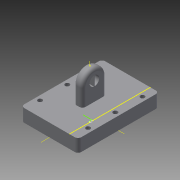
# Autodesk Inventor part: Camera holder with suppor final
Saved by Autodesk Inventor 2015 (Build 190159000, 159)
## iProperties
Created: 2016-05-06
Part Number: Camera holder with suppor final
Material: Generic
Document SubType Name: Modeling
Designer: Cristi
Density: 1 g/cm^3
Appearance: Default
Author: Cristi
Autodesk Inventor part; units mm, degrees
ref_plane "YZ Plane" through (0, 0, 0) normal (1, 0, 0) x (0, 1, 0)
ref_plane "XZ Plane" through (0, 0, 0) normal (0, 1, 0) x (-1, 0, 0)
ref_plane "XY Plane" through (0, 0, 0) normal (0, 0, 1) x (1, 0, 0)
sketch "Sketch1" plane through (0, 0, 0) normal (0, 0, 1) x (1, 0, 0)
  point P0 (0, 0)
sketch "Sketch2" plane through (0, 0, 0) normal (0, 1, 0) x (-1, 0, 0)
  line L0 (-17.8, 25.3) -> (-17.8, -25.3)
  line L1 (-17.8, -25.3) -> (-12.3, -25.3)
  line L2 (-12.3, -25.3) -> (-12.3, 25.3)
  line L3 (-12.3, 25.3) -> (-17.8, 25.3)
  circle A0 centre (-15, 16.2) radius 1.35
  circle A1 centre (-15, -0.8) radius 1.35
  circle A2 centre (-15, -17.8) radius 1.35
  point P0 (0, 0)
  point P1 (-17.8, 0)
  dimension "d0" = 50.6
  dimension "d1" = 5.5
  dimension "d2" = 2.8
  dimension "d3" = 2.7
  dimension "d4" = 9.1
  dimension "d5" = 2.7
  dimension "d6" = 2.7
  dimension "d7" = 17
  dimension "d8" = 17
  constraints: 8 end point, 3 centre point, 3 perpendicular, 2 vertical alignment, 1 midpoint, 1 vertical
  measures "d0" distance of L0.start L0.end
  measures "d1" distance of L0.end L1.end
  measures "d2" distance from line of L0 A0.centre
  measures "d3" diameter of A0
  measures "d4" distance from line of L3 A0.centre
  measures "d5" diameter of A1
  measures "d6" diameter of A2
  measures "d7" distance of A1.centre A2.centre
  measures "d8" distance of A0.centre A1.centre
extrude "Extrusion1" add sketch "Sketch2" along normal blind 8
sketch "Sketch3" plane through (12.3, 0, -25.3) normal (-1, 0, 0) x (0, 0, 1)
  line L0 (0, 8) -> (50.6, 8)
  line L1 (50.6, 8) -> (0, 8) projected
  line L2 (50.6, 8) -> (50.6, 5)
  line L3 (50.6, 0) -> (50.6, 8) projected
  line L4 (50.6, 5) -> (0, 5)
  line L5 (0, 0) -> (0, 8) projected
  point P0 (25.3, 0)
  dimension "d11" = 3
  constraints: 6 end point, 2 point on line, 1 collinear, 1 perpendicular
  measures "d11" distance of L0.end L2.end
extrude "Extrusion2" add sketch "Sketch3" along normal blind 12.3
mirror "Mirror1" about plane through (0, 0, 0) normal (1, 0, 0) of "Extrusion1", "Extrusion2"
sketch "Sketch4" plane through (0, 8, 0) normal (0, 1, 0) x (1, 0, 0)
  point P0 (0, 0)
sketch "Sketch5" plane through (0, 8, 0) normal (0, 1, 0) x (1, 0, 0)
  line L0 (-2.75, -7.5) -> (-2.75, 7.5)
  line L1 (-2.75, 7.5) -> (2.75, 7.5)
  line L2 (2.75, 7.5) -> (2.75, -7.5)
  line L3 (2.75, -7.5) -> (-2.75, -7.5)
  point P0 (0, 0)
  point P1 (-2.75, 0)
  point P2 (0, 7.5)
  dimension "d14" = 15
  dimension "d15" = 5.5
  constraints: 8 end point, 3 perpendicular, 2 midpoint, 1 horizontal alignment, 1 vertical, 1 vertical alignment
  measures "d14" distance of L0.start L0.end
  measures "d15" distance of L0.end L1.end
extrude "Extrusion3" add sketch "Sketch5" along normal blind 18
sketch "Sketch6" plane through (0, 26, 0) normal (0, 1, 0) x (1, 0, 0)
  point P0 (0, 0)
sketch "Sketch7" plane through (-2.75, 8, -7.5) normal (-1, 0, 0) x (0, 0, 1)
  point P0 (7.5, -8)
sketch "Sketch8" plane through (-2.75, 8, -7.5) normal (-1, 0, 0) x (0, 0, 1)
  circle A0 centre (7.5, 11.35) radius 3
  line L0 (0, 18) -> (15, 18) projected
  point P0 (7.5, -8)
  point P1 (7.5, 18)
  dimension "d18" = 6
  dimension "d19" = 6.65
  constraints: 1 centre point, 1 midpoint, 1 vertical alignment
  measures "d18" diameter of A0
  measures "d19" distance of point (7.5, 18) A0.centre
extrude "Extrusion4" cut sketch "Sketch8" against normal through all
fillet "Fillet1" radius 7.5 1 edges at (0, 26, 7.5)
fillet "Fillet2" radius 7.5 1 edges at (0, 26, -7.5)
sketch "Sketch9" plane through (12.3, 5, -25.3) normal (0, -1, 0) x (1, 0, 0)
  point P0 (-12.3, 25.3)
sketch "Sketch11" plane through (0, 8, 0) normal (0, 1, 0) x (1, 0, 0)
  line L0 (6.1515, -10.5742) -> (11.6515, -10.5742)
  line L1 (12.3, 25.3) -> (12.3, -25.3) projected
  line L2 (11.6515, -10.5742) -> (11.6515, -12.5742)
  point P0 (0, 0)
  dimension "d35" = 2
  constraints: 4 end point, 2 perpendicular
  measures "d35" distance of L0.end L2.end
sketch "Sketch12" plane through (-2.75, 8, -7.5) normal (-1, 0, 0) x (0, 0, 1)
  point P0 (7.5, -8)
sketch "Sketch14" plane through (2.75, 8, 7.5) normal (1, 0, 0) x (0, 0, -1)
  line L0 (7.25, 14.7235) -> (7.75, 14.7235)
  line L1 (7.75, 14.7235) -> (7.75, 7.9993)
  line L2 (7.75, 7.9993) -> (7.25, 7.9993)
  line L3 (7.25, 7.9993) -> (7.25, 14.7235)
  point P0 (7.5, -8)
  dimension "d40" = 0.5
  constraints: 8 end point, 3 perpendicular, 1 horizontal
  measures "d40" distance of L0.start L0.end
extrude "Extrusion7" add sketch "Sketch14" against normal up to surface (5.5 mm away)
fillet "Fillet3" radius 2 1 edges at (17.8, 4, 25.3)
fillet "Fillet4" radius 2 1 edges at (17.8, 4, -25.3)
fillet "Fillet5" radius 2 1 edges at (-17.8, 4, 25.3)
fillet "Fillet6" radius 2 1 edges at (-17.8, 4, -25.3)
fillet "Fillet7" radius 2 3 edges at (-2.75, 13.25, -7.5) (-2.75, 23.8033, 5.3033) (-2.75, 13.25, 7.5)
fillet "Fillet8" radius 2 3 edges at (2.75, 13.25, -7.5) (2.75, 23.8033, 5.3033) (2.75, 13.25, 7.5)
sketch "Sketch15" plane through (12.3, 5, -25.3) normal (0, -1, 0) x (1, 0, 0)
  line L0 (0, 0) -> (-24.6, 0)
  line L1 (0, 0) -> (-24.6, 0)
  line L2 (-24.6, 0) -> (-24.6, 0.5)
  line L3 (-24.6, 50.6) -> (-24.6, 0)
  line L4 (-24.6, 0.5) -> (-20.08, 0.5)
  line L5 (-20.08, 0.5) -> (-20.08, 25.05)
  line L6 (-20.08, 25.05) -> (-24.6, 25.05)
  line L7 (-24.6, 25.05) -> (-24.6, 25.55)
  line L8 (-24.6, 25.55) -> (-20.08, 25.55)
  line L9 (-20.08, 25.55) -> (-20.08, 50.1)
  line L10 (-20.08, 50.1) -> (-24.6, 50.1)
  line L11 (-24.6, 50.1) -> (-24.6, 50.6)
  line L12 (-24.6, 50.6) -> (0, 50.6)
  line L13 (0, 50.6) -> (-24.6, 50.6)
  line L14 (0, 50.6) -> (0, 50.1)
  line L15 (0, 50.1) -> (-4.52, 50.1)
  line L16 (0, 50.1) -> (4.52, 50.1) construction
  line L17 (-4.52, 50.1) -> (-4.52, 25.55)
  line L18 (-4.52, 25.55) -> (0, 25.55)
  line L19 (0, 25.55) -> (0, 25.05)
  line L20 (0, 25.05) -> (-4.52, 25.05)
  line L21 (-4.52, 25.05) -> (-4.52, 0.5)
  line L22 (-4.52, 0.5) -> (0, 0.5)
  line L23 (0, 0.5) -> (0, 0)
  line L24 (-5.02, 0.5) -> (-9.54, 0.5)
  line L25 (-9.54, 0.5) -> (-9.54, 25.05)
  line L26 (-9.54, 25.05) -> (-5.02, 25.05)
  line L27 (-5.02, 25.05) -> (-5.02, 0.5)
  line L28 (-5.02, 25.55) -> (-9.54, 25.55)
  line L29 (-9.54, 25.55) -> (-9.54, 50.1)
  line L30 (-9.54, 50.1) -> (-5.02, 50.1)
  line L31 (-5.02, 50.1) -> (-5.02, 25.55)
  line L32 (-10.04, 0.5) -> (-14.56, 0.5)
  line L33 (-14.56, 0.5) -> (-14.56, 25.05)
  line L34 (-14.56, 25.05) -> (-10.04, 25.05)
  line L35 (-10.04, 0.5) -> (-10.04, 25.05)
  line L36 (-10.04, 25.55) -> (-14.56, 25.55)
  line L37 (-10.04, 25.55) -> (-14.56, 25.55)
  line L38 (-14.56, 25.55) -> (-14.56, 50.1)
  line L39 (-14.56, 50.1) -> (-10.04, 50.1)
  line L40 (-10.04, 50.1) -> (-10.04, 25.55)
  line L41 (-15.06, 0.5) -> (-19.58, 0.5)
  line L42 (-19.58, 0.5) -> (-19.58, 25.05)
  line L43 (-19.58, 25.05) -> (-15.06, 25.05)
  line L44 (-15.06, 25.05) -> (-15.06, 0.5)
  line L45 (-15.06, 25.55) -> (-19.58, 25.55)
  line L46 (-19.58, 25.55) -> (-19.58, 50.1)
  line L47 (-19.58, 50.1) -> (-15.06, 50.1)
  line L48 (-15.06, 50.1) -> (-15.06, 25.55)
  line L49 (-15.06, 30.8) -> (-15.06, 25.55)
  line L50 (-15.06, 25.05) -> (-15.06, 19.8)
  line L51 (0, 0.5) -> (0, 0)
  line L52 (0, 25.55) -> (0, 25.05)
  line L53 (0, 50.6) -> (0, 50.1)
  line L54 (0, 0) -> (0, 50.6) projected
  line L55 (-24.6, 50.6) -> (-24.6, 50.1)
  line L56 (-24.6, 25.55) -> (-24.6, 25.05)
  line L57 (-24.6, 0.5) -> (-24.6, 0)
  point P0 (-12.3, 25.3)
  dimension "d49" = 0.5
  dimension "d51" = 24.55
  dimension "d52" = 0.5
  dimension "d53" = 24.55
  dimension "d55" = 180
  dimension "d65" = 0.5
  dimension "d66" = 4.52
  dimension "d67" = 0.5
  dimension "d68" = 4.52
  dimension "d69" = 0.5
  dimension "d70" = 4.52
  dimension "d71" = 0.5
  dimension "d72" = 4.52
  constraints: 114 end point, 20 horizontal alignment, 20 point on line, 14 horizontal, 9 vertical, 7 vertical alignment, 4 collinear, 2 perpendicular
  measures "d49" distance of L0.end L2.end
  measures "d51" distance of L4.end L5.end
  measures "d52" distance of L6.end L7.end
  measures "d53" distance of L8.end L9.end
  measures "d55" angle of L15 L16
  measures "d65" distance between parallel lines of L31 L17
  measures "d66" distance of L29.end L30.end
  measures "d67" distance between parallel lines of L40 L29
  measures "d68" distance of L39.end L38.end
  measures "d69" distance between parallel lines of L38 L48
  measures "d70" distance between parallel lines of L48 L46
  measures "d71" distance between parallel lines of L46 L9
  measures "d72" distance between parallel lines of L3 L9
extrude "Extrusion8" add sketch "Sketch15" along normal up to surface (5 mm away) contours L0 L2 L4 L5 L6 L3 L8 L9 L10 L12 L14 L15 L17 L18 L19 L20 L21 L22 L23
ref_plane "Work Plane1" through (0, 0, 0) normal (1, 0, 0) x (0, 1, 0)
body "Solid1"
